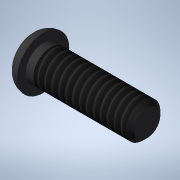
# Autodesk Inventor part: SNZS-M2-6
Saved by Autodesk Inventor 2021 (Build 250183000, 183)
## iProperties
Created: 2025-05-23
Part Number: SNZS-M2-6
Material: Generic
Catalog Web Link: www.cadenas.de
Description: SNZS-Pan Head Machine Screw for Precision Instruments
Vendor: NBK
Document SubType Name: Modeling
Designer: psAdmin
Manufacturer: NBK
Mass: 0.0217573 g
Surface Area: 0.590362 cm^2
Volume: 0.0217573 cm^3
Density: 1 g/cm^3
Appearance: PSOLRGB-175-175-175
Category: PARTsolutions
Company: NBK
Title: SNZS-M2-6
Author: Cadenas PARTsolutions
Comments: Pan Head Machine Screw for Precision Instruments
PSOL_IDENT_0: {$CADENAS_DATA/23d-libs/nbk/e_nedzi_com/miniature_screws/snzs.prj},157 {VTYP=3D},{NB=SNZS-M2-6},{LIN
PSOL_IDENT_1: A=SNZS-M2-6},{NN=SNZS},{DATE=22.05.2025 01:11:18},{GEOMDATE=12.07.2022 05:41:24},{VERSION=},{LINEID=
PSOL_IDENT_2: 400},{WBVAR=},{WBNUMERIC=}  {NB=SNZS-M2-6},{LINA=SNZS-M2-6},{KT=DUMMY},{CN=SNZS-M2-6},{M=M2},{L=6.0}
PSOL_IDENT_3: ,{D1=3.0},{L1=0.60},{A=0.00},{MT=0.220},{MASS=0.18},{NDM=2},{KDM=1.509},{VER=2}
NB: SNZS-M2-6
NN: SNZS
NT: Pan Head Machine Screw for Precision Instruments
NBSYN: $CN.
LINA: SNZS-M2-6
CATALOG: NBK (Nabeya Bi-tech Kaisha
CN: SNZS-M2-6
M: M2
L: 6
D1: 3
L1: 0.6
A: 0
SUPPLIER: NBK
ARTICLENO: SNZS-M2-6
BOMINFO: SNZS-M2-6
CREATOR: CADENAS GmbH
Autodesk Inventor part; units mm, degrees
ref_plane "YZ Plane" through (0, 0, 0) normal (1, 0, 0) x (0, 1, 0)
ref_plane "XZ Plane" through (0, 0, 0) normal (0, 1, 0) x (-1, 0, 0)
ref_plane "XY Plane" through (0, 0, 0) normal (0, 0, 1) x (1, 0, 0)
sketch "Sketch_1" plane through (0, 0, 0) normal (0, 0, 1) x (1, 0, 0)
  line L0 (6, 0) -> (-0.6, 0)
  line L1 (-0.6, 0) -> (-0.6, 1.2)
  arc A0 (0, 1.5) -> (-0.6, 1.2) centre (0, 0.75) ccw
  line L2 (0, 1.5) -> (0, 1)
  line L3 (0, 1) -> (5.7545, 1)
  line L4 (5.7545, 1) -> (6, 0.7545)
  line L5 (6, 0.7545) -> (6, 0)
  line L6 (6, 0) -> (-0.6, 0)
  constraints: 14 end point, 2 point on circle, 1 centre point
revolve "Revolution1" add sketch "Sketch_1" angle 360 about axis through (6, 0, 0) along (1, 0, 0)
thread "Thread1" size "M2x0.4" class "6g" standard "ISO Metric profile" length 5.3293
sketch "Sketch_2" plane through (0, 0, 0) normal (0, 0, 1) x (1, 0, 0)
  line L0 (-0.6, -0.9) -> (0.3, -0.45)
  line L1 (0.3, -0.45) -> (0.45, 0)
  line L2 (0.45, 0) -> (0.3, 0.45)
  line L3 (0.3, 0.45) -> (-0.6, 0.9)
  line L4 (-0.6, 0.9) -> (-0.6, -0.9)
  constraints: 10 end point
extrude "Extrusion1" cut sketch "Sketch_2" along normal mid plane 0.3
sketch "Sketch_3" plane through (0, 0, 0) normal (0, 1, 0) x (-1, 0, 0)
  line L0 (0.6, 0.9) -> (-0.3, 0.45)
  line L1 (-0.3, 0.45) -> (-0.45, 0)
  line L2 (-0.45, 0) -> (-0.3, -0.45)
  line L3 (-0.3, -0.45) -> (0.6, -0.9)
  line L4 (0.6, -0.9) -> (0.6, 0.9)
  constraints: 10 end point
extrude "Extrusion2" cut sketch "Sketch_3" along normal mid plane 0.3
body "Solid1"
